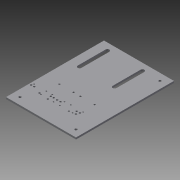
# Autodesk Inventor part: bottomLayer
Saved by Autodesk Inventor 2014 (Build 180170000, 170)
## iProperties
Created: 2014-10-04
Part Number: bottomLayer
Material: Generic
Document SubType Name: Modeling
Designer: Rachel
Density: 1 g/cm^3
Appearance: Default
Author: Rachel
Autodesk Inventor part; units mm, degrees
ref_plane "YZ Plane" through (0, 0, 0) normal (1, 0, 0) x (0, 1, 0)
ref_plane "XZ Plane" through (0, 0, 0) normal (0, 1, 0) x (-1, 0, 0)
ref_plane "XY Plane" through (0, 0, 0) normal (0, 0, 1) x (1, 0, 0)
sketch "Sketch1" plane through (0, 0, 0) normal (0, 1, 0) x (-1, 0, 0)
  line L0 (-63.5, 57.15) -> (63.5, 57.15)
  line L1 (63.5, 57.15) -> (63.5, -57.15)
  line L2 (63.5, -57.15) -> (-63.5, -57.15)
  line L3 (-63.5, -57.15) -> (-63.5, 57.15)
  line L4 (-63.5, 57.15) -> (63.5, -57.15) construction
  line L5 (63.5, 57.15) -> (-63.5, -57.15) construction
  line L6 (63.5, -57.15) -> (-38.1, -57.15)
  line L7 (-38.1, -57.15) -> (-38.1, -120.65)
  line L8 (-38.1, -120.65) -> (63.5, -120.65)
  line L9 (63.5, -120.65) -> (63.5, -57.15)
  line L10 (-38.1, -57.15) -> (-63.5, -57.15)
  line L11 (-63.5, -57.15) -> (-63.5, -120.65)
  line L12 (-63.5, -120.65) -> (-38.1, -120.65)
  line L13 (-38.1, -120.65) -> (-38.1, -57.15)
  point P0 (0, 0)
  dimension "d9" = 12.7
  dimension "d0" = 127
  dimension "d1" = 114.3
  dimension "d2" = 63.5
  dimension "d3" = 101.6
  constraints: 28 end point, 6 parallel, 3 horizontal, 3 perpendicular, 2 midpoint
  measures "d0" distance of L1.end L2.end
  measures "d1" distance of L0.end L1.end
  measures "d2" distance of L8.end L1.end
  measures "d3" distance of L7.end L8.end
extrude "Extrusion1" add sketch "Sketch1" along normal blind 3.175 contours L0 L1 L2 L3 | L9 L8 L7 L2
sketch "Sketch12" plane through (0, 3.175, 0) normal (0, 1, 0) x (1, 0, 0)
  line L0 (38.1, 57.15) -> (63.5, 57.15)
  line L1 (63.5, 57.15) -> (63.5, 120.65)
  line L2 (63.5, 120.65) -> (38.1, 120.65)
  line L3 (38.1, 120.65) -> (38.1, 57.15)
  point P0 (0, 0)
  dimension "d9" = 12.7
  constraints: 8 end point, 2 parallel, 1 horizontal, 1 perpendicular
extrude "Extrusion3" add sketch "Sketch12" against normal blind 3.175
sketch "Sketch2" plane through (0, 3.175, 0) normal (0, 1, 0) x (1, 0, 0)
  line L0 (-63.5, 120.65) -> (-63.5, -57.15) projected
  line L1 (-63.5, -57.15) -> (63.5, -57.15) projected
  line L2 (63.5, -57.15) -> (63.5, 57.15) projected
  line L3 (63.5, 57.15) -> (38.1, 57.15) projected
  line L4 (38.1, 57.15) -> (-63.5, 57.15) construction
  line L5 (-63.5, 57.15) -> (-63.5, -44.45) construction
  line L6 (-63.5, -44.45) -> (38.1, -44.45) construction
  line L7 (38.1, -44.45) -> (38.1, 57.15) construction
  line L8 (50.8, 57.15) -> (50.8, -57.15) construction
  line L9 (-63.5, -44.45) -> (63.5, -44.45) construction
  point P0 (0, 0)
  point P1 (50.8, -44.45)
  point P2 (50.8, 44.45)
  point P3 (-50.8, -44.45)
  dimension "d7" = 101.6
  dimension "d8" = 101.6
  dimension "d9" = 12.7
  dimension "d10" = 12.7
  dimension "d11" = 12.7
  constraints: 12 end point, 8 point on line, 4 perpendicular, 2 parallel, 1 horizontal, 1 midpoint
  measures "d7" distance of L5.end L6.end
  measures "d8" distance of L6.end L3.end
  measures "d9" distance between parallel lines of L1 L9
  measures "d10" distance from line of L0 point (-50.8, -44.45)
  measures "d11" distance from line of L3 point (50.8, 44.45)
hole "Hole1" at (50.8, 3.175, 44.45) at (-50.8, 3.175, 44.45) direction (0, -1, 0) diameter 4.191 end through all
sketch "Sketch3" plane through (0, 3.175, 0) normal (0, 1, 0) x (1, 0, 0)
  line L0 (38.1, 57.15) -> (38.1, 120.65) projected
  line L1 (38.1, 120.65) -> (-63.5, 120.65) projected
  line L2 (19.05, 107.95) -> (19.05, 57.15) construction
  line L3 (15.621, 107.95) -> (15.621, 57.15)
  line L4 (22.479, 57.15) -> (22.479, 107.95)
  arc A0 (22.479, 107.95) -> (15.621, 107.95) centre (19.05, 107.95) ccw
  arc A1 (15.621, 57.15) -> (22.479, 57.15) centre (19.05, 57.15) ccw
  line L5 (-12.7, 120.65) -> (-12.7, 57.15) construction
  line L6 (-44.45, 107.95) -> (-44.45, 57.15) construction
  line L7 (-41.021, 107.95) -> (-41.021, 57.15)
  line L8 (-47.879, 57.15) -> (-47.879, 107.95)
  arc A2 (-41.021, 107.95) -> (-47.879, 107.95) centre (-44.45, 107.95) ccw
  arc A3 (-47.879, 57.15) -> (-41.021, 57.15) centre (-44.45, 57.15) ccw
  point P0 (0, 0)
  point P1 (19.05, 82.55)
  point P2 (-44.45, 82.55)
  dimension "d19" = 6.858
  dimension "d20" = 19.05
  dimension "d21" = 12.7
  dimension "d22" = 50.8
  constraints: 18 end point, 8 point on circle, 7 symmetric about line, 4 centre point, 4 tangent, 3 parallel, 2 midpoint, 2 other
  measures "d19" diameter of A1
  measures "d20" distance between parallel lines of L0 L2
  measures "d21" distance from line of L1 L2.start
  measures "d22" distance of L2.start L2.end
extrude "Extrusion2" cut sketch "Sketch3" against normal through all
sketch "Sketch4" plane through (0, 3.175, 0) normal (0, 1, 0) x (1, 0, 0)
  arc A0 (15.621, 57.15) -> (22.479, 57.15) centre (19.05, 57.15) ccw projected
  line L0 (15.621, 57.15) -> (15.621, 107.95) projected
  arc A1 (22.479, 107.95) -> (15.621, 107.95) centre (19.05, 107.95) ccw projected
  line L1 (22.479, 107.95) -> (22.479, 57.15) projected
  arc A2 (-41.021, 107.95) -> (-47.879, 107.95) centre (-44.45, 107.95) ccw projected
  line L2 (-41.021, 107.95) -> (-41.021, 57.15) projected
  arc A3 (-47.879, 57.15) -> (-41.021, 57.15) centre (-44.45, 57.15) ccw projected
  line L3 (-47.879, 57.15) -> (-47.879, 107.95) projected
  circle A4 centre (50.8, 44.45) radius 3.2385 projected
  circle A5 centre (50.8, -44.45) radius 2.0955 projected
  circle A6 centre (-50.8, -44.45) radius 2.0955 projected
  line L4 (38.1, 57.15) -> (38.1, 120.65) projected
  line L5 (38.1, 120.65) -> (-63.5, 120.65) projected
  line L6 (-63.5, 120.65) -> (-63.5, -57.15) projected
  line L7 (-63.5, -57.15) -> (63.5, -57.15) projected
  line L8 (63.5, -57.15) -> (63.5, 57.15) projected
  line L9 (63.5, 57.15) -> (38.1, 57.15) projected
  line L10 (38.1, 57.15) -> (38.1, -57.15) construction
  line L11 (-63.5, -31.75) -> (63.5, -31.75) construction
  line L12 (-63.5, -25.4) -> (63.5, -25.4) construction
  line L13 (31.75, 53.1705) -> (31.75, -25.4) construction
  point P0 (0, 0)
  dimension "d9" = 12.7
  dimension "d25" = 25.4
  dimension "d156" = 31.75
  dimension "d157" = 31.75
  constraints: 8 end point, 6 point on line, 4 perpendicular
  measures "d25" distance between parallel lines of L7 L11
  measures "d156" distance between parallel lines of L7 L12
  measures "d157" distance between parallel lines of L8 L13
sketch "battery buzzer/ SmartSensorPowered" plane through (0, 3.175, 0) normal (0, 1, 0) x (1, 0, 0)
  line L0 (31.75, -12.7) -> (5.08, -12.7)
  line L1 (5.08, -12.7) -> (5.08, 34.29)
  line L2 (5.08, 34.29) -> (31.75, 34.29)
  line L3 (31.75, 34.29) -> (31.75, -12.7)
  circle A0 centre (29.972, -10.668) radius 1.1913
  circle A1 centre (7.62, -10.668) radius 1.1913
  line L4 (-1.27, -12.7) -> (-27.94, -12.7)
  line L5 (-27.94, -12.7) -> (-27.94, 34.29)
  line L6 (-27.94, 34.29) -> (-1.27, 34.29)
  line L7 (-1.27, 34.29) -> (-1.27, -12.7)
  circle A2 centre (-3.048, -11.2367) radius 1.1913
  circle A3 centre (-25.4, -11.2367) radius 1.1913
  line L8 (-34.29, -12.7) -> (-60.96, -12.7)
  line L9 (-60.96, -12.7) -> (-60.96, 34.29)
  line L10 (-60.96, 34.29) -> (-34.29, 34.29)
  line L11 (-34.29, 34.29) -> (-34.29, -12.7)
  circle A4 centre (-36.068, -11.2367) radius 1.1913
  circle A5 centre (-58.42, -11.2367) radius 1.1913
  line L12 (-63.5, -57.15) -> (63.5, -57.15) projected
  dimension "d9" = 12.7
  dimension "d242" = 26.67
  dimension "d248" = 46.99
  dimension "d251" = 2.3825
  dimension "d257" = 1.778
  dimension "d258" = 2.032
  dimension "d259" = 2.032
  dimension "d266" = 2.54
  dimension "d284" = 6.35
  dimension "d295" = 44.45
  constraints: 24 end point, 6 centre point, 3 perpendicular
  measures "d242" distance between parallel lines of L3 L1
  measures "d248" distance between parallel lines of L0 L2
  measures "d251" diameter of A0
  measures "d257" distance from line of L3 A0.centre
  measures "d258" distance from line of L0 A0.centre
  measures "d259" distance from line of L0 A1.centre
  measures "d266" distance from line of L1 A1.centre
  measures "d284" distance of L0.end L4.start
  measures "d295" distance between parallel lines of L12 L0
sketch "controller" plane through (0, 3.175, 0) normal (0, 1, 0) x (1, 0, 0)
  line L0 (-63.5, 120.65) -> (-63.5, -57.15) projected
  line L1 (63.5, -57.15) -> (63.5, 57.15) projected
  line L2 (-63.5, -57.15) -> (-63.5, -19.05) construction
  line L3 (-63.5, -57.15) -> (-63.5, -25.4) construction
  line L4 (-63.5, -25.4) -> (63.5, -25.4) construction
  line L5 (31.75, -25.4) -> (31.75, 57.15) construction
  line L6 (31.75, -25.4) -> (-44.45, -25.4)
  line L7 (-44.45, -25.4) -> (-44.45, 50.8)
  line L8 (-44.45, 50.8) -> (31.75, 50.8)
  line L9 (31.75, 50.8) -> (31.75, -25.4)
  circle A0 centre (26.67, -20.32) radius 1.651
  circle A1 centre (-39.37, -20.32) radius 1.651
  circle A2 centre (26.67, 45.72) radius 1.651
  circle A3 centre (-39.37, 45.72) radius 1.651
  point P0 (0, 0)
  dimension "d9" = 12.7
  dimension "d46" = 76.2
  dimension "d47" = 76.2
  dimension "d108" = 3.302
  dimension "d109" = 3.302
  dimension "d110" = 3.302
  dimension "d111" = 3.302
  dimension "d112" = 5.08
  dimension "d113" = 5.08
  dimension "d114" = 5.08
  dimension "d115" = 5.08
  dimension "d116" = 5.08
  dimension "d117" = 5.08
  dimension "d118" = 5.08
  dimension "d119" = 5.08
  constraints: 16 end point, 6 point on line, 4 centre point, 2 perpendicular, 1 collinear, 1 parallel
  measures "d46" distance of L5.start L6.end
  measures "d47" distance of L6.end L7.end
  measures "d108" diameter of A0
  measures "d109" diameter of A1
  measures "d110" diameter of A2
  measures "d111" diameter of A3
  measures "d112" distance from line of L9 A0.centre
  measures "d113" distance from line of L6 A0.centre
  measures "d114" distance from line of L4 A1.centre
  measures "d115" distance from line of L7 A1.centre
  measures "d116" distance from line of L5 A2.centre
  measures "d117" distance from line of L8 A2.centre
  measures "d118" distance from line of L8 A3.centre
  measures "d119" distance from line of L7 A3.centre
sketch "grizzly_bear" plane through (0, 3.175, 0) normal (0, 1, 0) x (1, 0, 0)
  line L0 (-63.5, 120.65) -> (-63.5, -57.15) projected
  line L1 (-63.5, -17.78) -> (63.5, -17.78) construction
  line L2 (31.75, -17.78) -> (-9.525, -17.78)
  line L3 (-15.875, -17.78) -> (-57.15, -17.78)
  line L4 (-57.15, -17.78) -> (-57.15, 58.42)
  line L5 (-57.15, 58.42) -> (-15.875, 58.42)
  line L6 (-15.875, 58.42) -> (-15.875, -17.78)
  line L7 (31.75, -17.78) -> (31.75, 58.42)
  line L8 (31.75, 58.42) -> (-9.525, 58.42)
  line L9 (-9.525, 58.42) -> (-9.525, -17.78)
  line L10 (63.5, 57.15) -> (63.5, 50.8) construction
  circle A0 centre (28.575, -14.986) radius 1.651
  circle A1 centre (-6.731, -14.986) radius 1.651
  circle A2 centre (28.575, 55.626) radius 1.651
  line L11 (63.5, -57.15) -> (63.5, 57.15) projected
  circle A3 centre (-19.05, -14.986) radius 1.651
  circle A4 centre (-54.356, -14.986) radius 1.651
  line L12 (-63.5, -25.4) -> (63.5, -25.4) construction
  point P0 (0, 0)
  point P1 (-15.875, -17.78)
  point P2 (-57.15, -17.78)
  dimension "d9" = 12.7
  dimension "d38" = 41.275
  dimension "d39" = 6.35
  dimension "d41" = 76.2
  dimension "d120" = 3.302
  dimension "d121" = 3.175
  dimension "d122" = 2.794
  dimension "d123" = 3.302
  dimension "d124" = 2.794
  dimension "d125" = 2.794
  dimension "d126" = 3.302
  dimension "d127" = 2.794
  dimension "d128" = 3.175
  dimension "d286" = 7.62
  constraints: 22 end point, 6 point on line, 5 centre point, 3 perpendicular, 2 parallel
  measures "d38" distance of L2.start L2.end
  measures "d39" distance of L2.end L3.start
  measures "d41" distance of L3.end L4.end
  measures "d120" diameter of A0
  measures "d121" distance from line of L7 A0.centre
  measures "d122" distance from line of L2 A0.centre
  measures "d123" diameter of A1
  measures "d124" distance from line of L2 A1.centre
  measures "d125" distance from line of L9 A1.centre
  measures "d126" diameter of A2
  measures "d127" distance from line of L8 A2.centre
  measures "d128" distance from line of L7 A2.centre
  measures "d286" distance from line of L12 L2.start
sketch "koala_bear" plane through (0, 3.175, 0) normal (0, 1, 0) x (1, 0, 0)
  line L0 (-63.5, 120.65) -> (-63.5, -57.15) projected
  line L1 (-63.5, -57.15) -> (63.5, -57.15) projected
  line L2 (63.5, -57.15) -> (63.5, 57.15) projected
  line L3 (-63.5, -25.4) -> (63.5, -25.4) construction
  line L4 (31.75, -57.15) -> (31.75, 57.15) construction
  line L5 (31.75, -25.4) -> (-0.127, -25.4)
  line L6 (-0.127, -25.4) -> (-0.127, 14.605)
  line L7 (-0.127, 14.605) -> (31.75, 14.605)
  line L8 (31.75, -25.4) -> (31.75, 14.605)
  line L9 (-6.477, -25.4) -> (-6.477, 14.605)
  line L10 (-6.477, 14.605) -> (-38.354, 14.605)
  line L11 (-38.354, 14.605) -> (-38.354, -25.4)
  line L12 (-6.477, -25.4) -> (-38.354, -25.4)
  circle A0 centre (28.702, 11.557) radius 1.524
  circle A1 centre (2.921, 11.557) radius 1.524
  circle A2 centre (2.921, -4.572) radius 1.524
  circle A3 centre (15.748, -22.225) radius 1.524
  circle A4 centre (-22.479, -22.225) radius 1.524
  circle A5 centre (-35.306, 11.557) radius 1.524
  circle A6 centre (-9.525, 11.557) radius 1.524
  point P0 (0, 0)
  dimension "d9" = 12.7
  dimension "d58" = 31.877
  dimension "d59" = 40.005
  dimension "d145" = 3.048
  dimension "d146" = 3.048
  dimension "d147" = 3.048
  dimension "d148" = 3.048
  dimension "d149" = 3.048
  dimension "d150" = 3.048
  dimension "d151" = 3.048
  dimension "d152" = 19.177
  dimension "d153" = 3.048
  dimension "d154" = 3.175
  dimension "d155" = 16.002
  constraints: 20 end point, 9 point on line, 7 centre point, 6 perpendicular, 2 parallel, 1 collinear
  measures "d58" distance of L5.start L5.end
  measures "d59" distance of L5.end L6.end
  measures "d145" diameter of A0
  measures "d146" distance from line of L8 A0.centre
  measures "d147" distance from line of L7 A0.centre
  measures "d148" diameter of A1
  measures "d149" distance from line of L6 A1.centre
  measures "d150" distance from line of L7 A1.centre
  measures "d151" diameter of A2
  measures "d152" distance from line of L7 A2.centre
  measures "d153" diameter of A3
  measures "d154" distance from line of L3 A3.centre
  measures "d155" distance from line of L8 A3.centre
sketch "smartsensor" plane through (0, 3.175, 0) normal (0, 1, 0) x (1, 0, 0)
  line L0 (-63.5, 120.65) -> (-63.5, -57.15) projected
  line L1 (63.5, -57.15) -> (63.5, 57.15) projected
  line L2 (-63.5, -25.4) -> (63.5, -25.4) construction
  line L3 (31.75, 54.3858) -> (31.75, -25.4) construction
  line L4 (24.13, -25.4) -> (-3.81, -25.4)
  line L5 (-3.81, -25.4) -> (-3.81, 7.62)
  line L6 (-3.81, 7.62) -> (24.13, 7.62)
  line L7 (24.13, 7.62) -> (24.13, -25.4)
  line L8 (-10.16, -25.4) -> (-38.1, -25.4)
  line L9 (-38.1, -25.4) -> (-38.1, 7.62)
  line L10 (-38.1, 7.62) -> (-10.16, 7.62)
  line L11 (-10.16, 7.62) -> (-10.16, -25.4)
  circle A0 centre (21.59, -21.59) radius 1.1913
  circle A1 centre (17.78, -21.59) radius 1.1913
  circle A2 centre (13.97, -21.59) radius 1.1913
  circle A3 centre (10.16, -21.59) radius 1.1913
  circle A4 centre (6.35, -21.59) radius 1.1913
  circle A5 centre (2.54, -21.59) radius 1.1913
  circle A6 centre (-1.27, -21.59) radius 1.1913
  circle A7 centre (-12.7, -21.59) radius 1.1913
  circle A8 centre (-16.51, -21.59) radius 1.1913
  circle A9 centre (-20.32, -21.59) radius 1.1913
  circle A10 centre (-24.13, -21.59) radius 1.1913
  circle A11 centre (-27.94, -21.59) radius 1.1913
  circle A12 centre (-31.75, -21.59) radius 1.1913
  circle A13 centre (-35.56, -21.59) radius 1.1913
  point P0 (0, 0)
  dimension "d9" = 12.7
  dimension "d64" = 27.94
  dimension "d65" = 33.02
  dimension "d129" = 2.3825
  dimension "d131" = 2.54
  dimension "d137" = 3.81
  dimension "d138" = 3.81
  dimension "d139" = 3.81
  dimension "d140" = 3.81
  dimension "d141" = 3.81
  dimension "d143" = 3.81
  dimension "d144" = 2.54
  dimension "d194" = 7.62
  dimension "d287" = 3.81
  constraints: 20 end point, 14 centre point, 5 perpendicular, 3 parallel, 2 point on line, 1 collinear
  measures "d64" distance of L4.start L4.end
  measures "d65" distance of L4.end L5.end
  measures "d129" diameter of A0
  measures "d131" distance from line of L7 A0.centre
  measures "d137" distance of A1.centre A0.centre
  measures "d138" distance of A2.centre A1.centre
  measures "d139" distance of A3.centre A2.centre
  measures "d140" distance of A4.centre A3.centre
  measures "d141" distance of A5.centre A4.centre
  measures "d143" distance of A5.centre A6.centre
  measures "d144" distance from line of L5 A6.centre
  measures "d194" distance between parallel lines of L3 L7
  measures "d287" distance from line of L4 A0.centre
sketch "team_flag" plane through (0, 3.175, 0) normal (0, 1, 0) x (1, 0, 0)
  line L0 (-63.5, 120.65) -> (-63.5, -57.15) projected
  line L1 (63.5, -57.15) -> (63.5, 57.15) projected
  line L2 (31.75, 51.8358) -> (31.75, -17.78) construction
  line L3 (25.4, -17.78) -> (-15.24, -17.78)
  line L4 (-15.24, -17.78) -> (-15.24, 22.86)
  line L5 (-15.24, 22.86) -> (25.4, 22.86)
  line L6 (25.4, 22.86) -> (25.4, -17.78)
  line L7 (-21.59, 22.86) -> (-21.59, -17.78)
  line L8 (-21.59, 22.86) -> (-62.23, 22.86)
  line L9 (-62.23, 22.86) -> (-62.23, -17.78)
  line L10 (-62.23, -17.78) -> (-21.59, -17.78)
  circle A0 centre (22.86, 20.32) radius 1.651
  circle A1 centre (-12.7, 20.32) radius 1.651
  circle A2 centre (-12.7, -15.24) radius 1.651
  circle A3 centre (22.86, -15.24) radius 1.651
  line L11 (-63.5, -25.4) -> (63.5, -25.4) construction
  circle A4 centre (-24.13, 20.32) radius 1.651
  circle A5 centre (-59.69, 20.32) radius 1.651
  circle A6 centre (-59.69, -15.24) radius 1.651
  circle A7 centre (-24.13, -15.24) radius 1.651
  point P0 (0, 0)
  point P1 (-21.59, -17.78)
  point P2 (-62.23, -17.78)
  point P3 (-62.23, 22.86)
  point P4 (-21.59, 22.86)
  dimension "d9" = 12.7
  dimension "d78" = 40.64
  dimension "d81" = 40.64
  dimension "d83" = 3.302
  dimension "d84" = 2.54
  dimension "d85" = 2.54
  dimension "d86" = 3.302
  dimension "d89" = 3.302
  dimension "d90" = 3.302
  dimension "d95" = 2.54
  dimension "d96" = 2.54
  dimension "d99" = 2.54
  dimension "d100" = 2.54
  dimension "d187" = 7.62
  dimension "d188" = 6.35
  dimension "d195" = 2.54
  constraints: 20 end point, 8 centre point, 3 perpendicular, 2 point on line, 1 parallel
  measures "d78" distance of L4.end L5.end
  measures "d81" distance between parallel lines of L3 L5
  measures "d83" diameter of A0
  measures "d84" distance from line of L6 A0.centre
  measures "d85" distance from line of L5 A0.centre
  measures "d86" diameter of A1
  measures "d89" diameter of A2
  measures "d90" diameter of A3
  measures "d95" distance from line of L5 A1.centre
  measures "d96" distance from line of L3 A3.centre
  measures "d99" distance from line of L4 A2.centre
  measures "d100" distance from line of L4 A1.centre
  measures "d187" distance between parallel lines of L11 L3
  measures "d188" distance between parallel lines of L6 L2
  measures "d195" distance from line of L6 A3.centre
hole "Hole2" at (29.972, 3.175, 10.668) at (7.62, 3.175, 10.668) at (-3.048, 3.175, 11.2367) at (-25.4, 3.175, 11.2367) at (-36.068, 3.175, 11.2367) at (-58.42, 3.175, 11.2367) direction (0, -1, 0) diameter 2.3876 end through all
hole "Hole3" at (-54.356, 3.175, 14.986) at (-19.05, 3.175, 14.986) at (-6.731, 3.175, 14.986) at (28.575, 3.175, 14.986) direction (0, -1, 0) diameter 3.302 end through all
hole "Hole4" at (22.86, 3.175, 15.24) at (-12.7, 3.175, 15.24) at (-24.13, 3.175, 15.24) at (-59.69, 3.175, 15.24) direction (0, -1, 0) diameter 3.302 end through all
hole "Hole5" at (26.67, 3.175, 20.32) at (-39.37, 3.175, 20.32) direction (0, -1, 0) diameter 3.302 end through all
hole "Hole6" at (21.59, 3.175, 21.59) at (-1.27, 3.175, 21.59) at (-12.7, 3.175, 21.59) at (-35.56, 3.175, 21.59) direction (0, -1, 0) diameter 2.3825 end through all
hole "Hole7" at (-35.306, 3.175, -11.557) at (2.921, 3.175, -11.557) at (-22.479, 3.175, 22.225) at (15.748, 3.175, 22.225) at (-9.525, 3.175, -11.557) at (28.702, 3.175, -11.557) direction (0, -1, 0) diameter 3.048 end through all
sketch "Sketch13" plane through (0, 3.175, 0) normal (0, 1, 0) x (1, 0, 0)
  point P0 (0, 0)
  point P1 (50.8, 107.95)
  dimension "d9" = 12.7
hole "Hole8" at (50.8, 3.175, -107.95) direction (0, -1, 0) diameter 4.191 end through all
body "Solid1"
